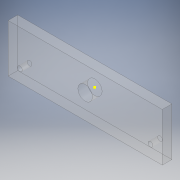
# Autodesk Inventor part: structural small
Saved by Autodesk Inventor 2018 (Build 220112000, 112)
## iProperties
Created: 2018-12-07
Part Number: structural small
Material: Polycarbonate, Clear
Document SubType Name: Modeling
Designer: Jayden
Density: 1.2 g/cm^3
Appearance: Polycarbonate - Clear
Author: Jayden
Autodesk Inventor part; units mm, degrees
note: some values were not read from the file. Chosen so that the rebuilt part matches the saved one: second side of "Extrusion1".
ref_plane "YZ Plane" through (0, 0, 0) normal (1, 0, 0) x (0, 1, 0)
ref_plane "XZ Plane" through (0, 0, 0) normal (0, 1, 0) x (-1, 0, 0)
ref_plane "XY Plane" through (0, 0, 0) normal (0, 0, 1) x (1, 0, 0)
sketch "Sketch1" plane through (0, 0, 0) normal (0, 0, 1) x (1, 0, 0)
  point P0 (0, 0)
sketch "Sketch2" plane through (0, 0, 0) normal (0, 0, 1) x (1, 0, 0)
  line L0 (-50.8, 15.875) -> (50.8, 15.875)
  line L1 (50.8, 15.875) -> (50.8, -15.875)
  line L2 (50.8, -15.875) -> (-50.8, -15.875)
  line L3 (-50.8, -15.875) -> (-50.8, 15.875)
  circle A0 centre (0, 0) radius 4.7625
  circle A1 centre (43, -7.8) radius 1.5875
  circle A2 centre (-43, -7.8) radius 1.5875
  dimension "d0" = 101.6
  dimension "d1" = 31.75
  dimension "d3" = 50.8
  dimension "d4" = 15.875
  dimension "d5" = 15.875
  dimension "d6" = 9.525
  dimension "d7" = 3.175
  dimension "d8" = 3.175
  dimension "d9" = 7.8
  dimension "d10" = 43
  dimension "d11" = 43
  dimension "d12" = 7.8
  constraints: 8 end point, 3 centre point, 2 parallel, 1 coincident, 1 horizontal, 1 perpendicular
  measures "d0" distance of L1.end L2.end
  measures "d1" distance of L0.end L1.end
  measures "d3" distance from line of L3 point (0, 0)
  measures "d4" distance from line of L2 point (0, 0)
  measures "d5" distance from line of point (0, 0) L0
  measures "d6" diameter of A0
  measures "d7" diameter of A1
  measures "d8" diameter of A2
  measures "d9" vertical distance of point (0, 0) A2.centre
  measures "d10" horizontal distance of A2.centre point (0, 0)
  measures "d11" horizontal distance of A1.centre point (0, 0)
  measures "d12" vertical distance of A1.centre point (0, 0)
extrude "Extrusion1" add sketch "Sketch2" along normal blind 6.35
body "Solid1"
